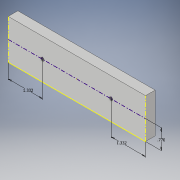
# Autodesk Inventor part: nmt_metalplate
Saved by Autodesk Inventor 2017 (Build 210142000, 142)
## iProperties
Created: 2017-02-18
Part Number: nmt_metalplate
Material: Generic
Document SubType Name: Modeling
Designer: Zara
Density: 1 g/cm^3
Appearance: Default
Author: Zara
Autodesk Inventor part; units mm, degrees
ref_plane "YZ Plane" through (0, 0, 0) normal (1, 0, 0) x (0, 1, 0)
ref_plane "XZ Plane" through (0, 0, 0) normal (0, 1, 0) x (-1, 0, 0)
ref_plane "XY Plane" through (0, 0, 0) normal (0, 0, 1) x (1, 0, 0)
sketch "Sketch1" plane through (0, 0, 0) normal (0, 0, 1) x (1, 0, 0)
  line L0 (-67.6402, -19.558) -> (67.6402, -19.558)
  line L1 (67.6402, -19.558) -> (67.6402, 19.558)
  line L2 (67.6402, 19.558) -> (-67.6402, 19.558)
  line L3 (-67.6402, 19.558) -> (-67.6402, -19.558)
  line L4 (-67.6402, -19.558) -> (67.6402, 19.558) construction
  line L5 (67.6402, -19.558) -> (-67.6402, 19.558) construction
  point P0 (0, 0)
  dimension "d0" = 135.2804
  dimension "d1" = 39.116
  constraints: 12 end point, 2 midpoint, 2 parallel, 1 horizontal, 1 perpendicular
  measures "d0" distance of L1.end L2.end
  measures "d1" distance of L0.end L1.end
extrude "Extrusion1" add sketch "Sketch1" along normal blind 9.525
sketch "Sketch2" plane through (0, 0, 9.525) normal (0, 0, 1) x (1, 0, 0)
  line L0 (-67.5894, 0) -> (67.7772, 0)
  line L1 (-67.6402, 19.558) -> (-67.6402, -19.558) projected
  line L2 (67.6402, -19.558) -> (67.6402, 19.558) projected
  line L3 (-67.6402, -19.558) -> (67.6402, -19.558) projected
  point P0 (0, 0)
  point P1 (-33.8074, 0)
  point P2 (33.8074, 0)
  dimension "d4" = 33.8328
  dimension "d5" = 33.8328
  dimension "d13" = 19.558
  constraints: 2 end point, 2 point on line, 1 horizontal
  measures "d4" distance from line of point (-33.807, 0) L1
  measures "d5" distance from line of point (33.807, 0) L2
  measures "d13" distance between parallel lines of L0 L3
hole "Hole1" at (-33.8074, 0, 9.525) at (33.8074, 0, 9.525) direction (0, 0, -1) diameter 3.2512 end through all
body "Solid1"
